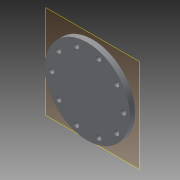
# Autodesk Inventor part: topPlate
Saved by Autodesk Inventor 2013 (Build 170138000, 138)
## iProperties
Created: 2013-02-05
Part Number: topPlate
Material: Polycarbonate, Clear
Document SubType Name: Modeling
Designer: Nano
Mass: 7.56399 g
Surface Area: 47.9868 cm^2
Volume: 6.30332 cm^3
Density: 1.2 g/cm^3
Author: Nano
Autodesk Inventor part; units mm, degrees
ref_plane "YZ Plane" through (0, 0, 0) normal (1, 0, 0) x (0, 1, 0)
ref_plane "XZ Plane" through (0, 0, 0) normal (0, 1, 0) x (-1, 0, 0)
ref_plane "XY Plane" through (0, 0, 0) normal (0, 0, 1) x (1, 0, 0)
ref_plane "Work Plane1" through (0, 0, 0) normal (0, 0, 1) x (1, 0, 0)
sketch "Sketch1" plane through (0, 0, 0) normal (0, 0, 1) x (1, 0, 0)
  circle A0 centre (0, 0) radius 25.6348 projected
  circle A1 centre (-6.7, 20.6205) radius 1.5875 projected
  circle A2 centre (6.7, 20.6205) radius 1.5875 projected
  circle A3 centre (17.5408, 12.7442) radius 1.5875 projected
  circle A4 centre (21.6817, 0) radius 1.5875 projected
  circle A5 centre (17.5408, -12.7442) radius 1.5875 projected
  circle A6 centre (6.7, -20.6205) radius 1.5875 projected
  circle A7 centre (-6.7, -20.6205) radius 1.5875 projected
  circle A8 centre (-17.5408, -12.7442) radius 1.5875 projected
  circle A9 centre (-21.6817, 0) radius 1.5875 projected
  circle A10 centre (-17.5408, 12.7442) radius 1.5875 projected
  point P0 (0, 0)
extrude "Extrusion1" add sketch "Sketch1" along normal blind 3.175
body "Solid1"
